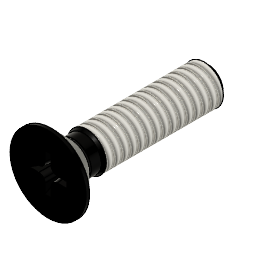
SplitKbBothSides (Autodesk Fusion 360 archive; units mm, degrees)
design "Countersunk Flat Head Screw PN-EN ISO 7046-1 - M2 x 8 - H Steel 4.6 Black"
description: Countersunk Flat Head Screw PN-EN ISO 7046-1 - M2 x 8 - H
part number: PN-EN ISO 7046-1 - M2 x 8 - H Steel 4.6 Black
Autodesk Fusion 360 part; units mm, degrees
sketch "Sketch1" plane through (0, 0, 0) normal (0, 1, 0) x (1, 0, 0)
  line L0 (0, -2.0773) -> (-1.9, -2.0773)
  line L1 (-1.9, -2.0773) -> (-1.9, -1.9)
  line L2 (-1.9, -1.9) -> (-0.8773, -0.8773)
  line L3 (-1, -0.0773) -> (-1, 5.9227)
  line L4 (-1, 5.9227) -> (0, 5.9227)
  line L5 (0, 5.9227) -> (0, -2.0773)
  line L6 (-0.8773, -0.2898) -> (-0.8773, -0.8773)
  line L7 (-1, -0.0773) -> (-0.8773, -0.2898)
  dimension "d9" = 2
  dimension "d11" = 3.8
  dimension "d71" = 1.2
  dimension "d72" = 1.7546
  dimension "d89" = 6
  dimension "d101" = 30
  dimension "d115" = 8
  dimension "d121" = 45
  constraint perpendicular L0 L1
  constraint vertical L3
  constraint perpendicular L3 L4
  constraint perpendicular L0 L5
  constraint collinear origin L0.start L4.end
  constraint horizontal L0
  constraint coincident L2.end L6.end
  constraint coincident L6 L7.end
  constraint coincident L6.start L7.end
  constraint coincident origin L2
  measures "d71" distance of L0 L2.end
  measures "d89" distance of L4 L3.start
  measures "d101" angle of L3 L7
  measures "d115" distance of L0.start L4
  measures "d121" angle of L2 L5
revolve "Revolve1" add sketch "Sketch1" angle 360 about axis through (0, 0, -5.9227) along (0, 0, 1) makes body 1
sketch "Sketch2" plane through (0, 0, 2.0773) normal (0, 0, 1) x (1, 0, 0)
  line L0 (-0.155, 0.155) -> (-0.95, 0.155)
  line L1 (-0.95, 0.155) -> (-0.95, -0.155)
  line L2 (-0.95, -0.155) -> (-0.155, -0.155)
  line L3 (0.155, -0.95) -> (0.155, -0.155)
  line L4 (-0.155, -0.95) -> (0.155, -0.95)
  line L5 (-0.155, -0.155) -> (-0.155, -0.95)
  line L6 (0.95, 0.155) -> (0.155, 0.155)
  line L7 (0.95, -0.155) -> (0.95, 0.155)
  line L8 (0.155, -0.155) -> (0.95, -0.155)
  line L9 (-0.155, 0.95) -> (-0.155, 0.155)
  line L10 (0.155, 0.95) -> (-0.155, 0.95)
  line L11 (0.155, 0.155) -> (0.155, 0.95)
  dimension "d111" = 360
  dimension "d117" = 1.9
  dimension "d122" = 0.31
  constraint horizontal L0
  constraint perpendicular L0 L1
  constraint vertical L0.start L2.end
  constraint coincident L0.start L9.end
  measures "d117" distance of L4.start L10
  measures "d122" distance of L0 L2
extrude "Extrude1" add sketch "Sketch2" against normal blind 1.2 draft -4 separate body makes body 2
draft "Draft1" angle -30 neutral plane through (0, 0, 2.0773) pull (0, 0, 1) 4 faces at (0.922, -0.0237, 1.6773) (0.0237, 0.922, 1.6773) (-0.922, 0.0237, 1.6773) (-0.0237, -0.922, 1.6773) on bodies 2
fillet "Fillet3" radius 0.31 4 edges at (0.113, 0.113, 1.4773) (0.113, -0.113, 1.4773) (-0.113, -0.113, 1.4773) (-0.113, 0.113, 1.4773) on bodies 2
combine "Combine1" operation cut target body 1 tool bodies 2
thread "Thread1" "ISO Metric profile 2.0 M2x0.4 M2x0.4 6g" major diameter 1.9335 minor diameter 1.478 pitch 0.4 angle 60 resizes the face on face at (-0.9988, 0.0498, -1.9227) on bodies 1
fillet "Fillet5" radius 0.2 1 edges at (-0.8179, 0.3172, 0.8773) on bodies 1
sketch "Sketch6" plane through (0, 0, 0) normal (0, 1, 0) x (1, 0, 0)
  line L0 (-0.7546, 5.9227) -> (-1.02, 5.9227)
  line L1 (-1.02, 5.9227) -> (-1.02, 5.6773)
  line L2 (-1.02, 5.6773) -> (-0.7546, 5.9227)
  line L3 (-1, 5.9227) -> (0, 5.9227)
  line L4 (0, 0) -> (0, 5.9227) construction
  dimension "d102" = 1.02
  dimension "d118" = 0.7546
  dimension "d119" = 0.2454
  constraint horizontal L0
  constraint perpendicular L0 L1
  constraint coincident L0.start L3
  constraint coincident L4.start origin
  constraint coincident L3.end L4.end
  measures "d102" distance of L4.start L1
  measures "d118" distance of L0.start L4
  measures "d119" distance of L0 L1.end
revolve "Revolve3" cut sketch "Sketch6" angle 360 about axis through (0, 0, 1.75) along (0, 0, 1) bodies 1
equation "d9 = adsk_nomdia"
equation "d11 = adsk_headdia"
equation "adsk_nomlen = 8.00 mm"
equation "adsk_headh = 1.20 mm"
equation "adsk_headdia = 3.80 mm"
equation "adsk_nomdia = 2.00 mm"
equation "adsk_headang = 90.00 deg"
equation "adsk_phildia = 1.90 mm"
equation "d31 = -adsk_phildepth"
equation "adsk_philwidth = 0.31 mm"
equation "adsk_phildepth = 1.20 mm"
equation "d71 = adsk_headh"
equation "d72 = adsk_shnkdia"
equation "adsk_shnkdia = 1.75462 mm"
equation "d89 = adsk_thrlen"
equation "adsk_thrlen = 6.00 mm"
equation "adsk_pitch1 = 0.40 mm"
equation "adsk_startlen = 0.24538 mm"
equation "adsk_midfillet = adsk_nomdia * 0.1"
equation "d96 = adsk_midfillet"
equation "d99 = ( adsk_shnkdia / 2 ) * tan(90 deg - adsk_headang / 2) + adsk_headh"
equation "d102 = adsk_nomdia * 0.51"
equation "adsk_endpointdia = 1.50924 mm"
equation "d114 = adsk_philwidth"
equation "d115 = adsk_nomlen"
equation "d117 = adsk_phildia"
equation "d118 = adsk_endpointdia / 2"
equation "d119 = adsk_startlen"
equation "d121 = adsk_headang * 0.5"
equation "d122 = adsk_philwidth"
